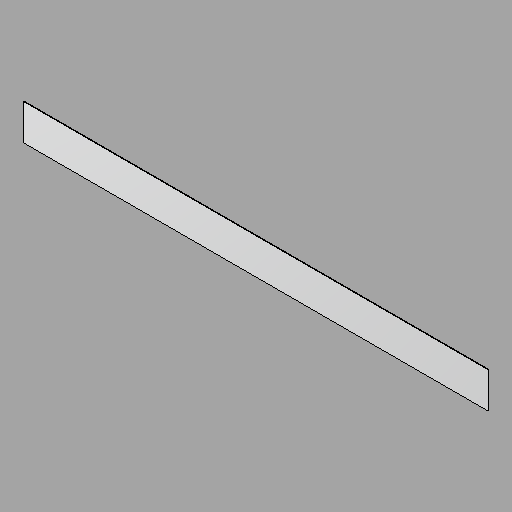
# Autodesk Inventor part: 板
Saved by Autodesk Inventor 2022 (Build 260153000, 153)
## iProperties
Created: 2021-07-07
Part Number: 板
Material: アルミニウム 6061
Document SubType Name: Modeling
Designer: nrz71
Density: 2.7 g/cm^3
Appearance: アルミニウム - フラット
Mass: 13.4719 g
Surface Area: 203.461 cm^2
Volume: 4.9896 cm^3
Author: nrz71
Autodesk Inventor part; units mm, degrees
ref_plane "YZ Plane" through (0, 0, 0) normal (1, 0, 0) x (0, 1, 0)
ref_plane "XZ Plane" through (0, 0, 0) normal (0, 1, 0) x (-1, 0, 0)
ref_plane "XY Plane" through (0, 0, 0) normal (0, 0, 1) x (1, 0, 0)
sketch "スケッチ1" plane through (0, 0, 0) normal (0, 0, 1) x (1, 0, 0)
  line L0 (-176, -2.5) -> (176, -2.5) projected
  line L1 (-175, -20.22) -> (-175, -2.5) projected
  line L2 (176, -20.22) -> (-176, -20.22) projected
  line L3 (175, -2.5) -> (175, -20.22) projected
  line L4 (-176, -25.22) -> (176, -25.22) projected
  line L5 (-180, -150) -> (-180, 5) projected
  line L6 (180, 5) -> (180, -150) projected
  line L7 (176, 2.5) -> (-176, 2.5) projected
  line L8 (180, 2.5) -> (-180, 2.5)
  line L9 (-180, 2.5) -> (-180, -25.22)
  line L10 (-180, -25.22) -> (180, -25.22)
  line L11 (180, -25.22) -> (180, 2.5)
  point P0 (0, 0)
  point P1 (180, -25.22)
  point P2 (-180, 2.5)
  constraints: 8 end point, 3 point on line, 2 parallel, 1 horizontal, 1 perpendicular
extrude "押し出し1" add sketch "スケッチ1" along normal blind 0.5 contours L0 L3 L2 L1 | L10 L5 L8 L7 L6 L4
